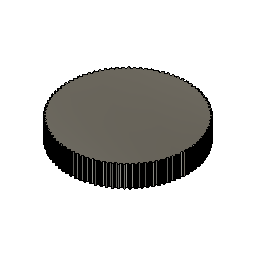
gear_89z (Autodesk Fusion 360 design; units mm, degrees)
Autodesk Fusion 360 part; units mm, degrees
sketch "Sketch1" plane through (0, 0, 0) normal (0, 0, 1) x (1, 0, 0) in component "gt2 pulley"
  circle A0 centre (0, 0) radius 28.3296 construction
  circle A1 centre (0, 0) radius 27.3256 construction
  line L0 (0, 0) -> (0, 28.3296) construction
  line L1 (0, 0) -> (0.9998, 28.3119) construction
  line L2 (0, 0) -> (1.4045, 28.2947) construction
  circle A2 centre (0, 0) radius 28.0756 construction
  arc A3 (0.397, 27.9397) -> (0.4752, 27.6414) centre (1.3919, 28.0411) ccw
  circle A4 centre (0, 0) radius 27.9256 construction
  arc A5 (0.2491, 28.0745) -> (0, 28.0756) centre (0, 0) ccw
  arc A6 (0.397, 27.9397) -> (0.2491, 28.0745) centre (0.2478, 27.9245) ccw
  arc A7 (0.4752, 27.6414) -> (0.9644, 27.3086) centre (0.9839, 27.8632) ccw
  arc A8 (0, 28.0756) -> (-0.2491, 28.0745) centre (0, 0) ccw
  arc A9 (-0.2491, 28.0745) -> (-0.397, 27.9397) centre (-0.2478, 27.9245) ccw
  arc A10 (-0.4752, 27.6414) -> (-0.397, 27.9397) centre (-1.3919, 28.0411) ccw
  arc A11 (-0.9642, 27.3086) -> (-0.4752, 27.6414) centre (-0.9839, 27.8632) ccw
  arc A12 (0.9644, 27.3086) -> (-0.9644, 27.3086) centre (0, 0) ccw
  point P0 (1.3919, 28.0411)
  point P1 (0, 28.0756)
  dimension "d18" = 56.6592
  dimension "d19" = 2.022
  dimension "d22" = 1.004
  dimension "d24" = 0.75
  dimension "d26" = 1
  dimension "d27" = 0.15
  dimension "d28" = 0.15
  dimension "d47" = 0.555
  dimension "d52" = 3.812
  constraint coincident A0.centre A1.centre
  constraint coincident A0 L0.end
  constraint vertical L0
  constraint coincident A0 L1.end
  constraint coincident A0 L2.end
  constraint concentric A1 A2
  constraint coincident A1 A7.end
  constraint coincident L1 A7.end
  constraint coincident A2 P0
  constraint coincident L2 P0
  constraint coincident P0 A3.centre
  constraint coincident A2 P1
  constraint coincident L0 P1
  constraint concentric A2 A4
  constraint coincident P1 A5.end
  constraint coincident A4 A6.centre
  constraint coincident A3.start A6.start
  constraint tangent A3 A6
  constraint tangent A3 A7
  constraint symmetric L0 A7.end A12.end
  constraint symmetric L0 A3.start A9.end
  constraint symmetric L0 A3.end A10.start
  constraint symmetric L0 A3 A10
  constraint symmetric L0 A5.start A8.end
  constraint symmetric L0 P1 A5.end
  constraint symmetric L0 A5 A8
  constraint symmetric L0 A6 A9
  constraint symmetric L0 A7 A11
  constraint coincident A1 A11.start
  constraint tangent A1 A7
  constraint coincident L1 A7.centre
  measures "d18" diameter of A0
  measures "d19" angle of L0 L1
  measures "d22" distance of A0 A1
  measures "d24" distance of A1 A2
  measures "d26" radius of A3
  measures "d27" distance of A2 A4
  measures "d28" radius of A6
  measures "d47" radius of A7
extrude "Extrude1" add sketch "Sketch1" along normal blind 10 makes body 1
pattern_circular "C-Pattern1" count 89 over 360 about axis through (0, 0, 1.75) along (0, 0, 1) of bodies 1 makes body 2 at (-2.0343, 27.2497, 6.6667) makes body 3 at (-3.1013, 27.149, 3.3333) makes body 4 at (-5.8488, 26.6923, 6.6667) makes body 5 at (-7.7171, 26.2132, 6.6667) makes body 6 at (-8.7391, 25.8905, 3.3333) makes body 7 at (-11.3292, 24.8664, 6.6667) makes body 8 at (-12.2956, 24.403, 3.3333) makes body 9 at (-15.2535, 22.672, 6.6667) makes body 10 at (-15.6074, 22.4298, 3.3333) makes body 11 at (-18.2922, 20.2998, 6.6667) makes body 12 at (-18.6085, 20.0102, 3.3333) makes body 13 at (-20.5488, 18.012, 6.6667) makes body 14 at (-21.7682, 16.5177, 6.6667) makes body 15 at (-23.2243, 14.3986, 6.6667) makes body 16 at (-23.876, 13.2899, 6.6667) makes body 17 at (-25.0194, 10.987, 6.6667) makes body 18 at (-25.1888, 10.5931, 3.3333) makes body 19 at (-25.8733, 8.7899, 6.6667) makes body 20 at (-26.77, 5.4821, 6.6667) makes body 21 at (-26.8527, 5.0614, 3.3333) makes body 22 at (-27.2751, 1.6603, 6.6667) makes body 23 at (-27.2978, 1.2321, 3.3333) makes body 24 at (-27.3167, -0.6965, 3.3333) makes body 25 at (-27.1995, -2.6217, 3.3333) makes body 26 at (-26.6574, -6.0057, 6.6667) makes body 27 at (-26.3453, -7.2533, 6.6667) makes body 28 at (-25.547, -9.6974, 6.6667) makes body 29 at (-25.0624, -10.8886, 6.6667) makes body 30 at (-23.9281, -13.196, 6.6667) makes body 31 at (-23.7181, -13.5699, 6.6667) makes body 32 at (-22.7018, -15.2091, 3.3333) makes body 33 at (-20.6195, -17.9311, 6.6667) makes body 34 at (-19.753, -18.8814, 6.6667) makes body 35 at (-17.8909, -20.6544, 6.6667) makes body 36 at (-17.5646, -20.9326, 3.3333) makes body 37 at (-15.3425, -22.6118, 6.6667) makes body 38 at (-14.444, -23.1961, 3.3333) makes body 39 at (-12.0077, -24.5459, 6.6667) makes body 40 at (-11.0359, -24.9979, 3.3333) makes body 41 at (-8.434, -25.9915, 6.6667) makes body 42 at (-7.4083, -26.3022, 3.3333) makes body 43 at (-5.5345, -26.7592, 3.3333) makes body 44 at (-2.1414, -27.2415, 6.6667) makes body 45 at (-0.2145, -27.3247, 6.6667) makes body 46 at (0.2143, -27.3247, 3.3333) makes body 47 at (3.633, -27.083, 6.6667) makes body 48 at (5.5343, -26.7593, 6.6667) makes body 49 at (7.4081, -26.3022, 6.6667) makes body 50 at (9.245, -25.7142, 6.6667) makes body 51 at (10.4446, -25.2507, 6.6667) makes body 52 at (11.4267, -24.8217, 3.3333) makes body 53 at (14.4439, -23.1962, 6.6667) makes body 54 at (16.0441, -22.1195, 6.6667) makes body 55 at (17.5644, -20.9327, 6.6667) makes body 56 at (17.8908, -20.6545, 3.3333) makes body 57 at (19.3031, -19.3411, 3.3333) makes body 58 at (20.6193, -17.9313, 3.3333) makes body 59 at (22.3376, -15.7392, 6.6667) makes body 60 at (22.9376, -14.8511, 6.6667) makes body 61 at (23.928, -13.1961, 3.3333) makes body 62 at (25.3116, -10.296, 6.6667) makes body 63 at (25.5469, -9.6975, 3.3333) makes body 64 at (26.1673, -7.8713, 3.3333) makes body 65 at (26.8327, -5.1667, 6.6667) makes body 66 at (27.0146, -4.1105, 3.3333) makes body 67 at (27.2927, -1.3392, 6.6667) makes body 68 at (27.3243, -0.2679, 3.3333) makes body 69 at (27.2096, 2.5149, 6.6667) makes body 70 at (26.8528, 5.0612, 6.6667) makes body 71 at (26.77, 5.482, 3.3333) makes body 72 at (26.073, 8.1785, 6.6667) makes body 73 at (25.4311, 9.9973, 6.6667) makes body 74 at (25.0195, 10.9869, 3.3333) makes body 75 at (24.1822, 12.7244, 3.3333) makes body 76 at (22.7613, 15.1199, 6.6667) makes body 77 at (22.0247, 16.1741, 6.6667) makes body 78 at (20.967, 17.5234, 3.3333) makes body 79 at (19.6787, 18.9588, 3.3333) makes body 80 at (18.2924, 20.2997, 3.3333) makes body 81 at (16.1309, 22.0563, 6.6667) makes body 82 at (15.2536, 22.6719, 3.3333) makes body 83 at (12.8665, 24.1069, 6.6667) makes body 84 at (11.9113, 24.5929, 3.3333) makes body 85 at (9.346, 25.6776, 6.6667) makes body 86 at (8.3319, 26.0244, 6.6667) makes body 87 at (6.4754, 26.5473, 3.3333) makes body 88 at (3.7394, 27.0685, 6.6667) makes body 89 at (1.8207, 27.2649, 6.6667)
sketch "Sketch2" plane through (0, 0, 10) normal (0, 0, 1) x (-1, 0, 0)
  arc A0 (-10.0314, -26.0798) -> (-9.9391, -26.2574) centre (-9.8861, -26.1171) ccw
  arc A1 (-9.9391, -26.2574) -> (-9.4717, -26.4296) centre (0, 0) ccw
  arc A2 (-9.4717, -26.4296) -> (-9.2863, -26.3543) centre (-9.4211, -26.2884) ccw
  arc A3 (-9.1098, -26.1014) -> (-9.2863, -26.3543) centre (-8.3878, -26.7933) ccw
  arc A4 (-8.5359, -25.9582) -> (-9.1098, -26.1014) centre (-8.7091, -26.4854) ccw
  arc A5 (-10.3456, -25.2914) -> (-8.5359, -25.9582) centre (0, 0) ccw
  arc A6 (-10.0016, -25.7729) -> (-10.3456, -25.2914) centre (-10.5557, -25.8051) ccw
  arc A7 (-10.0314, -26.0798) -> (-10.0016, -25.7729) centre (-10.9999, -25.831) ccw
  circle A8 centre (0, 0) radius 27.3256
  constraint concentric A1 A8
extrude "Extrude2" add sketch "Sketch2" against normal blind 10 contours A5 A8 bodies 1 2 3 4 5 6 7 8 9 10 11 12 13 14 15 16 17 18 19 20 21 22 23 24 25 26 27 28 29 30 31 32 33 34 35 36 37 38 39 40 41 42 43 44 45 46 47 48 49 50 51 52 53 54 55 56 57 58 59 60 61 62 63 64 65 66 67 68 69 70 71 72 73 74 75 76 77 78 79 80 81 82 83 84 85 86 87 88 89
extrude "Extrude4" [suppressed] in component "gt2 pulley"
pattern_circular "C-Pattern7" [suppressed] in component "gt2 pulley"
extrude "Extrude3" [suppressed] in component "gt2 pulley"
pattern_circular "C-Pattern6" [suppressed] in component "gt2 pulley"
extrude "Extrude2'" [suppressed] in component "gt2 pulley"
pattern_circular "C-Pattern5" [suppressed] in component "gt2 pulley"
extrude "Extrude1'" [suppressed] in component "gt2 pulley"
pattern_circular "C-Pattern4" [suppressed] in component "gt2 pulley"
pattern_circular "C-Pattern3" [suppressed] in component "gt2 pulley"
pattern_circular "C-Pattern2" [suppressed] in component "gt2 pulley"
pattern_circular "C-Pattern1'" [suppressed] in component "gt2 pulley"
copy_body "Body->Comp1" [suppressed] in component "Component"
copy_body "Body->Comp2" [suppressed] in component "Component'"
copy_body "Body->Comp3" [suppressed] in component "Component''"
copy_body "Body->Comp4" [suppressed] in component "Component'''"
copy_body "Body->Comp5" [suppressed] in component "Component''''"
copy_body "Body->Comp6" [suppressed] in component "Component'''''"
copy_body "Body->Comp7" [suppressed] in component "Component''''''"
copy_body "Body->Comp8" [suppressed] in component "Component'''''''"
copy_body "Body->Comp9" [suppressed] in component "Component''''''''"
copy_body "Body->Comp10" [suppressed] in component "Component'''''''''"
copy_body "Body->Comp11" [suppressed] in component "Component''''''''''"
copy_body "Body->Comp12" [suppressed] in component "Component'''''''''''"
copy_body "Body->Comp13" [suppressed] in component "Component''''''''''''"
copy_body "Body->Comp14" [suppressed] in component "Component'''''''''''''"
copy_body "Body->Comp15" [suppressed] in component "Component''''''''''''''"
copy_body "Body->Comp16" [suppressed] in component "Component'''''''''''''''"
copy_body "Body->Comp17" [suppressed] in component "Component''''''''''''''''"
copy_body "Body->Comp18" [suppressed] in component "Component'''''''''''''''''"
copy_body "Body->Comp19" [suppressed] in component "Component''''''''''''''''''"
copy_body "Body->Comp20" [suppressed] in component "Component'''''''''''''''''''"
component "gt2 pulley" placed x (1, 0, 0) y (0, 1, 0) z (0, 0, 1) at (0, 0, 0)
equation "NumTeeth = 89" comment "min 20"
equation "ToothPitch = 2 mm"
equation "PullyDia = NumTeeth * ToothPitch / PI"
equation "ToothAng = ( ( 360 / NumTeeth ) * 1 deg )"
equation "TransOffsetAngle = ToothAng * 0.2"
equation "Sholulder_Radius = 0.15 mm"
equation "Root_Radius = 0.555 mm"
equation "TransRadius = 1 mm"
equation "ToolHeight = 0.75 mm"
equation "PLD = 0.254 mm"
equation "d18 = PullyDia"
equation "d19 = ToothAng / 2"
equation "d22 = PLD + ToolHeight"
equation "d24 = ToolHeight"
equation "d26 = TransRadius"
equation "d27 = Sholulder_Radius"
equation "d31 = NumTeeth"
equation "d33 = NumTeeth"
equation "d35 = NumTeeth"
equation "d37 = NumTeeth"
equation "d41 = NumTeeth"
equation "d45 = NumTeeth"
equation "d47 = Root_Radius"
equation "d50 = NumTeeth"
